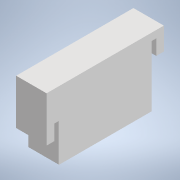
# Autodesk Inventor part: BumperFrameStandoff
Saved by Autodesk Inventor 2020 (Build 240168000, 168)
## iProperties
Created: 2020-03-12
Part Number: BumperFrameStandoff
Material: Generic
Document SubType Name: Modeling
Designer: srini
Density: 1 g/cm^3
Appearance: Default
Author: srini
Autodesk Inventor part; units mm, degrees
ref_plane "YZ Plane" through (0, 0, 0) normal (1, 0, 0) x (0, 1, 0)
ref_plane "XZ Plane" through (0, 0, 0) normal (0, 1, 0) x (-1, 0, 0)
ref_plane "XY Plane" through (0, 0, 0) normal (0, 0, 1) x (1, 0, 0)
sketch "Sketch1" plane through (0, 0, 0) normal (1, 0, 0) x (0, 1, 0)
  line L0 (92.1534, 119.6677) -> (119.9664, 119.6677) construction
  arc A0 (92.1534, 119.6677) -> (91.3914, 118.9057) centre (92.1534, 118.9057) ccw construction
  line L1 (91.3914, 118.9057) -> (91.3914, 42.1977) construction
  arc A1 (91.3914, 42.1977) -> (92.1534, 41.4357) centre (92.1534, 42.1977) ccw construction
  line L2 (139.0164, 41.4357) -> (92.1534, 41.4357) construction
  line L3 (148.5414, 119.3677) -> (92.1534, 119.3677)
  arc A2 (92.1534, 119.3677) -> (91.6914, 118.9057) centre (92.1534, 118.9057) ccw
  line L4 (91.6914, 118.9057) -> (91.6914, 42.1977)
  arc A3 (91.6914, 42.1977) -> (92.1534, 41.7357) centre (92.1534, 42.1977) ccw
  line L5 (92.1534, 41.7357) -> (148.5414, 41.7357)
  line L6 (148.5414, 119.3677) -> (148.5414, 41.7357)
  line L7 (142.1914, 41.4357) -> (142.1914, 38.2607) construction
  line L8 (123.1414, 122.8427) -> (123.1414, 119.6677) construction
  line L9 (119.9664, 122.8427) -> (123.1414, 122.8427) construction
  line L10 (142.1914, 38.2607) -> (139.0164, 38.2607) construction
  line L11 (123.4414, 119.3677) -> (148.5414, 119.3677)
  line L12 (148.5414, 119.3677) -> (148.5414, 123.1427)
  line L13 (148.5414, 123.1427) -> (123.4414, 123.1427)
  line L14 (123.4414, 123.1427) -> (123.4414, 119.3677)
  line L15 (148.5414, 123.1427) -> (110.7414, 123.1427)
  line L16 (110.7414, 123.1427) -> (110.7414, 129.4927)
  line L17 (110.7414, 129.4927) -> (148.5414, 129.4927)
  line L18 (148.5414, 129.4927) -> (148.5414, 123.1427)
  line L19 (142.4914, 41.7357) -> (148.5414, 41.7357)
  line L20 (148.5414, 41.7357) -> (148.5414, 37.9607)
  line L21 (148.5414, 37.9607) -> (142.4914, 37.9607)
  line L22 (142.4914, 37.9607) -> (142.4914, 41.7357)
  line L23 (148.5414, 37.9607) -> (129.7914, 37.9607)
  line L24 (129.7914, 37.9607) -> (129.7914, 31.6107)
  line L25 (129.7914, 31.6107) -> (148.5414, 31.6107)
  line L26 (148.5414, 31.6107) -> (148.5414, 37.9607)
  point P0 (0, 0)
  dimension "d0" = 0.3
  dimension "d1" = 6.35
  dimension "d2" = 0.3
  dimension "d3" = 0.3
  dimension "d4" = 0.3
  dimension "d5" = 0.3
  dimension "d6" = 6.35
  dimension "d7" = 6.35
  dimension "d8" = 12.7
  dimension "d9" = 12.7
  constraints: 40 end point, 8 parallel, 4 horizontal, 4 perpendicular, 4 point on circle, 2 centre point, 2 collinear, 2 point on line, 1 vertical, 4 other
  measures "d0" distance between parallel lines of L3 L0
  measures "d1" distance between parallel lines of L7 L6
  measures "d2" distance between parallel lines of L23 L10
  measures "d3" distance between parallel lines of L7 L22
  measures "d4" distance between parallel lines of L8 L14
  measures "d5" distance between parallel lines of L9 L15
  measures "d6" distance of L25.end L20.end
  measures "d7" distance of L17.end L12.end
  measures "d8" distance between parallel lines of L16 L14
  measures "d9" distance between parallel lines of L22 L24
extrude "Extrusion1" add sketch "Sketch1" along normal blind 25.4
equation "\"d2\" = d0"
equation "\"d3\" = d0"
equation "\"d4\" = d0"
equation "\"d5\" = d0"
body "Solid1"
